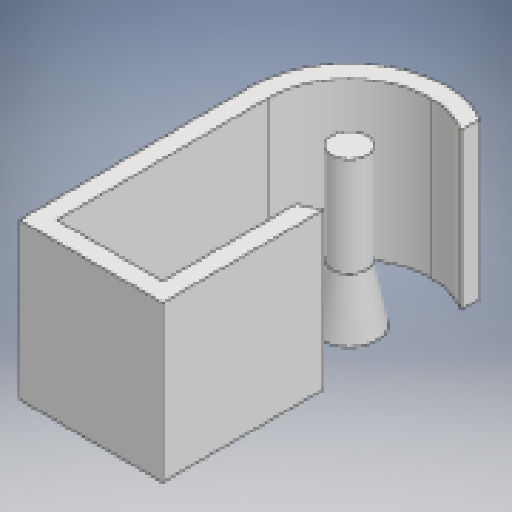
# Autodesk Inventor part: body
Saved by Autodesk Inventor 2025.2 (Build 292293000, 293)
## iProperties
Created: 2025-03-09
Part Number: body
Material: Generic
Document SubType Name: Modeling
Designer: Alex
Density: 1 g/cm^3
Appearance: Default
Author: Alex
Autodesk Inventor part; units mm, degrees
ref_plane "YZ Plane" through (0, 0, 0) normal (1, 0, 0) x (0, 1, 0)
ref_plane "XZ Plane" through (0, 0, 0) normal (0, 1, 0) x (-1, 0, 0)
ref_plane "XY Plane" through (0, 0, 0) normal (0, 0, 1) x (1, 0, 0)
sketch "Sketch1" plane through (0, 0, 0) normal (1, 0, 0) x (0, 1, 0)
  line L0 (0, 0) -> (0, -9.15) construction
  line L1 (0, -9.15) -> (9.0687, -2.8) construction
  line L2 (9.0687, -2.8) -> (9.0687, 0) construction
  line L3 (0, -9.15) -> (0, -29.4542) construction
  line L4 (0, 0) -> (49.8191, 0) construction
  line L5 (9.0687, 0) -> (0, 0)
  line L6 (9.0687, -2.8) -> (25.35, -2.8)
  line L7 (25.35, -2.8) -> (25.35, 0)
  line L8 (25.35, 0) -> (9.0687, 0)
  line L9 (9.0687, -2.8) -> (0, -4.3991)
  line L10 (0, 0) -> (0, -4.3991)
  dimension "d1" = 125
  dimension "d2" = 5.6
  dimension "d3" = 9.15
  dimension "d5" = 9.0687
  dimension "d6" = 25.35
  dimension "d8" = 80
  constraints: 22 end point, 3 collinear, 2 horizontal, 2 point on line, 2 vertical, 1 parallel, 1 perpendicular
  measures "d1" angle of L3 L1
  measures "d2" diameter of L1.end L4
  measures "d3" distance of L0.start L0.end
  measures "d5" distance of L0.start L2.end
  measures "d6" distance between parallel lines of L3 L7
  measures "d8" angle of L0 L9
revolve "Revolution1" add sketch "Sketch1" angle 360 about axis through (0, 0, 0) along (0, 1, 0)
sketch "Sketch2" plane through (0, 0, 0) normal (0, -1, 0) x (1, 0, 0)
  line L0 (6.9, -13.1) -> (-16.1, -13.1) construction
  line L1 (-16.1, -13.1) -> (-16.1, 36.9)
  line L2 (-16.1, 36.9) -> (6.9, 36.9)
  line L3 (6.9, 36.9) -> (6.9, -13.1) construction
  circle A0 centre (0, 0) radius 12.5 construction
  circle A1 centre (0, 0) radius 13 construction
  line L4 (6.9, -13.1) -> (6.9, -11.0177) construction
  line L5 (6.9, 36.9) -> (6.9, 11.0177)
  line L6 (0, -13.1) -> (0, -13) construction
  line L7 (3.9, 12.4012) -> (3.9, 33.9)
  line L8 (3.9, 33.9) -> (-13.1, 33.9)
  line L9 (-13.1, 33.9) -> (-13.1, 0)
  arc A2 (6.9, 11.0177) -> (3.9, 12.4012) centre (0, 0) ccw
  arc A3 (-13.1, 0) -> (0, -13.1) centre (0, 0) ccw
  line L10 (0, -13.1) -> (0, -16.1) construction
  line L11 (-13.1, 0) -> (-13, 0) construction
  circle A4 centre (0, 0) radius 2.8 projected
  line L12 (0, 0) -> (-13, 0) construction
  arc A5 (0, -13.1) -> (6.9, -11.0177) centre (0.1762, -1.2107) ccw
  line L13 (-13.1, 0) -> (-16.1, 0) construction
  arc A6 (-16.1, 0) -> (0, -16.1) centre (0, 0) ccw
  line L14 (6.9, -11.0177) -> (6.9, -14.0177)
  arc A7 (0, -16.1) -> (6.9, -14.0177) centre (0, -3.6267) ccw
  dimension "d9" = 25
  dimension "d10" = 0.5
  dimension "d11" = 3
  dimension "d12" = 3
  dimension "d13" = 3
  dimension "d15" = 3
  dimension "d16" = 23
  dimension "d18" = 0.1
  dimension "d19" = 0.1
  dimension "d22" = 3
  dimension "d23" = 11.8906
  dimension "d24" = 50
  constraints: 30 end point, 15 point on circle, 7 centre point, 5 perpendicular, 4 point on line, 4 tangent, 3 horizontal, 3 vertical, 2 parallel, 1 coincident, 1 concentric
  measures "d9" diameter of A0
  measures "d10" radial gap between concentric circles of A0 A1
  measures "d11" distance between parallel lines of L1 L9
  measures "d12" distance between parallel lines of L8 L2
  measures "d13" distance between parallel lines of L7 L3
  measures "d15" distance of L6.start L10.end
  measures "d16" distance of L0.start L0.end
  measures "d18" distance of L9.end L11.end
  measures "d19" distance of L6.start L6.end
  measures "d22" distance of L4.end L14.end
  measures "d23" radius of A5
  measures "d24" distance of L0.end L1.end
extrude "Extrusion1" add sketch "Sketch2" against normal up to surface (25.35 mm away) contours L1 L2 L5 A2 L7 L8 L9 A3 A5 L14 A7 A6
sketch "Sketch3" plane through (0, 0, 0) normal (0, -1, 0) x (1, 0, 0)
  line L0 (6.9, 11.0177) -> (6.9, 36.9) projected
  line L1 (6.9, 36.9) -> (-16.1, 36.9) projected
  line L2 (-16.1, 36.9) -> (-16.1, 0) projected
  arc A0 (-16.1, 0) -> (0, -16.1) centre (0, 0) ccw projected
  arc A1 (0, -16.1) -> (6.9, -14.0177) centre (0, -3.6267) ccw projected
  line L3 (6.9, -14.0177) -> (6.9, -11.0177) projected
  arc A2 (0, -13.1) -> (6.9, -11.0177) centre (0.1762, -1.2107) ccw construction
  line L4 (6.9, 11.0177) -> (6.9, -11.0177) construction
  arc A3 (6.9, -10.4177) -> (6.9, 10.4177) centre (-0.0081, 0) ccw construction
  arc A4 (6.9, -10.6569) -> (6.9, 10.6569) centre (-0.0081, 0) ccw
  line L5 (6.9, 0) -> (12.6919, 0) construction
  line L6 (6.9, -10.6569) -> (6.9, -11.0177)
  line L7 (6.9, 11.0177) -> (6.9, 10.6569)
  point P0 (0, 0)
  dimension "d29" = 12.5
  dimension "d30" = 0.2
  dimension "d31" = 0.6
  constraints: 8 end point, 5 point on circle, 4 point on line, 2 centre point, 1 collinear, 1 horizontal, 1 midpoint, 1 vertical
  measures "d29" radius of A3
  measures "d30" radial gap between concentric circles of A3 A4
  measures "d31" distance of L3.end A3.start
extrude "Extrusion2" add sketch "Sketch3" along normal blind 3
mirror "Mirror1" about plane through (0, 25.35, 0) normal (0, 1, 0) of "Extrusion1", "Extrusion2", "Revolution1"
body "Solid1"
